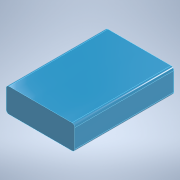
# Autodesk Inventor part: baterka
Saved by Autodesk Inventor 2022 (Build 260153000, 153)
## iProperties
Created: 2022-02-10
Part Number: baterka
Material: Generic
Document SubType Name: Modeling
Designer: matys
Density: 1 g/cm^3
Appearance: Sky Blue Dark
Author: matys
Autodesk Inventor part; units mm, degrees
ref_plane "YZ Plane" through (0, 0, 0) normal (1, 0, 0) x (0, 1, 0)
ref_plane "XZ Plane" through (0, 0, 0) normal (0, 1, 0) x (-1, 0, 0)
ref_plane "XY Plane" through (0, 0, 0) normal (0, 0, 1) x (1, 0, 0)
sketch "Sketch1" plane through (0, 0, 0) normal (0, 1, 0) x (-1, 0, 0)
  line L0 (0, 0) -> (0, -69)
  line L1 (0, -69) -> (48, -69)
  line L2 (48, -69) -> (48, 0)
  line L3 (48, 0) -> (0, 0)
  dimension "d0" = 69
  dimension "d1" = 48
  constraints: 8 end point, 3 perpendicular, 1 vertical
  measures "d0" distance of L0.start L0.end
  measures "d1" distance of L0.end L1.end
extrude "Extrusion1" add sketch "Sketch1" along normal blind 17
fillet "Fillet1" radius 2 4 edges at (0, 17, -34.5) (-48, 17, -34.5) (0, 0, -34.5) (-48, 0, -34.5)
body "Solid1"
